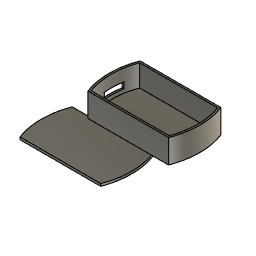
Earthquake Detector_Case v1 (Autodesk Fusion 360 design; units mm, degrees)
Autodesk Fusion 360 part; units mm, degrees
sketch "Sketch1" plane through (0, 0, 0) normal (0, 0, 1) x (1, 0, 0)
  line L0 (0, 0) -> (170, 0)
  arc A0 (0, 0) -> (0, -110) centre (145, -55) ccw
  line L1 (170, -110) -> (0, -110)
  arc A1 (170, -110) -> (170, 0) centre (25, -55) ccw
  constraint coincident L0.start A0.start
  constraint horizontal L0
  constraint horizontal L1
extrude "Extrude1" add sketch "Sketch1" along normal blind 55 makes body 1
shell "Shell1" thickness 4 removed faces 0 bodies 1
ref_plane "WorkPlane1" through (85, -55, 50) normal (0, 0, 1) x (1, 0, 0)
split "Split1" by plane through (85, -55, 50) normal (0, 0, 1) bodies 1 makes body 2 at (53.4423, -51.255, 55)
move_body "Move1" bodies 2 to x (1, 0, 0) y (0, 1, 0) z (0, 0, 1) at (-143.139, 0, -160.3978)
sketch "Sketch2" plane through (0, 0, 0) normal (1, 0, 0) x (0, 1, 0)
  line L0 (-70, 12) -> (-30, 12)
  line L1 (-30, 12) -> (-30, 25)
  line L2 (-30, 25) -> (-70, 25)
  line L3 (-70, 25) -> (-70, 12)
  constraint horizontal L0
  constraint vertical L1
  constraint horizontal L2
  constraint vertical L3
extrude "Extrude2" cut sketch "Sketch2" against normal blind 20 bodies 1
